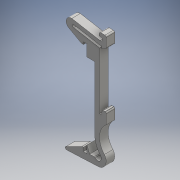
# Autodesk Inventor part: raspDinClipmmv3
Saved by Autodesk Inventor 2016 (Build 200138000, 138)
## iProperties
Created: 2016-08-27
Part Number: raspDinClipmmv3
Material: Generic
Document SubType Name: Modeling
Designer: Thetheos
Density: 1 g/cm^3
Appearance: Default
Author: Thetheos
Autodesk Inventor part; units mm, degrees
ref_plane "YZ Plane" through (0, 0, 0) normal (1, 0, 0) x (0, 1, 0)
ref_plane "XZ Plane" through (0, 0, 0) normal (0, 1, 0) x (-1, 0, 0)
ref_plane "XY Plane" through (0, 0, 0) normal (0, 0, 1) x (1, 0, 0)
sketch "Sketch1" plane through (0, 0, 0) normal (0, 1, 0) x (-1, 0, 0)
  arc A0 (-159.7794, 702.6597) -> (-160.5669, 701.8721) centre (-159.7794, 701.8721) ccw
  line L0 (-155.7462, 702.6597) -> (-155.7462, 704.2667)
  line L1 (-155.7462, 704.2667) -> (-153.5139, 704.2667)
  line L2 (-153.5139, 704.2667) -> (-153.5139, 702.7873)
  line L3 (-153.5139, 702.7873) -> (-152.617, 702.7873)
  arc A1 (-164.1836, 648.4268) -> (-160.5669, 657.8731) centre (-174.7114, 657.8731) ccw
  line L4 (-160.5669, 657.8731) -> (-160.5669, 701.8721)
  arc A2 (-160.1794, 645.8656) -> (-160.7583, 645.6139) centre (-160.1783, 645.0714) ccw
  arc A3 (-164.1836, 648.4268) -> (-160.7583, 645.6139) centre (-162.4137, 647.0901) ccw
  line L5 (-155.7462, 648) -> (-155.7462, 645.3343)
  line L6 (-155.7462, 645.3343) -> (-153.4959, 645.3343)
  line L7 (-153.4959, 645.3343) -> (-153.4959, 647.6194)
  arc A4 (-143.0505, 641.0266) -> (-142.8499, 642.7649) centre (-143.1474, 641.9185) ccw
  line L8 (-163.0481, 641.9081) -> (-143.0505, 641.0266)
  arc A5 (-166.527, 650.2868) -> (-163.0481, 641.9081) centre (-162.4027, 647.0877) ccw
  arc A6 (-166.527, 650.2868) -> (-167.6435, 666.7468) centre (-174.834, 657.9912) ccw
  line L9 (-166.9993, 673.5601) -> (-165.874, 673.5549)
  arc A7 (-165.1258, 673.0171) -> (-165.874, 673.5549) centre (-165.8807, 672.7563) ccw
  arc A8 (-163.8545, 670.6656) -> (-163.5889, 670.9316) centre (-163.8582, 670.9349) ccw
  line L10 (-163.5889, 706.0242) -> (-163.5889, 706.0613)
  line L11 (-163.5889, 706.0613) -> (-147.5669, 708.9022)
  arc A9 (-147.5669, 708.9022) -> (-147.8271, 710.4852) centre (-147.6086, 709.7082) ccw
  line L12 (-147.8271, 710.4852) -> (-163.5899, 707.6952)
  line L13 (-163.5899, 707.6952) -> (-164.9831, 707.6944)
  line L14 (-164.9831, 707.6944) -> (-164.9826, 706.5463)
  arc A10 (-165.396, 706.3271) -> (-164.9826, 706.5463) centre (-165.2521, 706.5552) ccw
  line L15 (-165.396, 706.3271) -> (-167.2486, 707.3943)
  arc A11 (-167.6628, 708.0983) -> (-167.2486, 707.3943) centre (-166.8615, 708.0959) ccw
  line L16 (-167.6628, 708.0983) -> (-167.6658, 713.6939)
  arc A12 (-166.8627, 714.4991) -> (-167.6658, 713.6939) centre (-166.8611, 713.6943) ccw
  line L17 (-166.8627, 714.4991) -> (-164.1837, 714.5007)
  arc A13 (-163.3795, 713.6976) -> (-164.1837, 714.5007) centre (-164.1848, 713.6954) ccw
  line L18 (-163.3795, 713.6976) -> (-163.3787, 712.3581)
  line L19 (-163.3787, 712.3581) -> (-165.5216, 711.9789)
  line L20 (-165.5216, 711.9789) -> (-165.5215, 711.7106)
  arc A14 (-165.5215, 711.7106) -> (-163.8456, 710.1095) centre (-163.9177, 711.7116) ccw
  line L21 (-163.8456, 710.1095) -> (-146.318, 713.1891)
  arc A15 (-144.6103, 707.1134) -> (-146.318, 713.1891) centre (-146.0422, 709.9888) ccw
  arc A16 (-152.617, 702.7873) -> (-152.2474, 702.8795) centre (-152.6236, 703.6003) ccw
  line L22 (-155.7462, 702.6597) -> (-155.7462, 700.1597)
  line L23 (-155.7462, 700.1597) -> (-156.9462, 700.1597)
  line L24 (-156.9462, 700.1597) -> (-157.7628, 702.6597)
  line L25 (-157.7628, 702.6597) -> (-159.7794, 702.6597)
  line L26 (-155.7462, 648) -> (-155.7462, 650)
  line L27 (-155.7462, 650) -> (-157.3545, 645.8656)
  line L28 (-157.3545, 645.8656) -> (-160.1794, 645.8656)
  line L29 (-144.6103, 707.1134) -> (-152.2474, 702.8795)
  line L30 (-152.5619, 647.6194) -> (-153.4959, 647.6194)
  line L31 (-163.8545, 670.6656) -> (-164.6545, 670.6656)
  arc A17 (-164.8084, 670.8401) -> (-164.6545, 670.6656) centre (-164.6322, 670.8403) ccw
  line L32 (-163.5889, 670.9316) -> (-163.5889, 706.0613)
  line L33 (-164.8084, 670.8401) -> (-165.1258, 673.0171)
  line L34 (-167.6435, 666.7468) -> (-167.6666, 672.6833)
  line L35 (-166.9993, 673.5601) -> (-167.2486, 673.5601)
  arc A18 (-167.2486, 673.5601) -> (-167.6666, 672.6833) centre (-166.547, 672.6876) ccw
  line L36 (-142.8499, 642.7649) -> (-152.5619, 647.6194)
  point P0 (-160.5669, 683.588)
  dimension "d2" = 43.999
  dimension "d6" = 2.5
  dimension "d7" = 1.2
  dimension "d8" = 2
  dimension "d18" = 0.8
  dimension "d20" = 2.2
  constraints: 74 end point, 38 point on circle, 19 centre point, 6 perpendicular, 5 horizontal, 2 tangent, 2 vertical
  measures "d2" distance of L4.start L4.end
  measures "d6" distance of L0.start L22.end
  measures "d7" distance of L22.end L23.end
  measures "d8" distance of L5.start L26.end
  measures "d18" distance of L31.start L31.end
  measures "d20" distance of L33.start L33.end
extrude "Extrusion1" add sketch "Sketch1" along normal blind 5.3
sketch "Sketch2" plane through (0, 0, 0) normal (0, -1, 0) x (1, 0, 0)
  line L0 (156.9462, 700.1597) -> (155.7462, 700.1597) projected
  line L1 (155.7462, 700.1597) -> (155.7462, 697.1597)
  line L2 (155.7462, 697.1597) -> (160.5669, 697.1597)
  line L3 (160.5669, 657.8731) -> (160.5669, 701.8721) projected
  line L4 (160.5669, 697.1597) -> (160.5783, 702.6397)
  line L5 (160.5783, 702.6397) -> (155.7462, 704.198)
  line L6 (155.7462, 704.198) -> (155.7462, 700.1597)
  point P0 (0, 0)
  dimension "d9" = 3
  constraints: 10 end point, 1 collinear, 1 perpendicular, 1 point on line, 1 vertical
  measures "d9" distance of L0.end L1.end
extrude "Extrusion2" add sketch "Sketch2" against normal blind 5.3
sketch "Sketch3" plane through (155.7462, 0, 704.2667) normal (-1, 0, 0) x (0, 0, 1)
  circle A0 centre (-4.5576, 2.65) radius 1.25
  line L0 (-7.107, 5.3) -> (0, 5.3) projected
  line L1 (0, 0) -> (-7.107, 0) projected
  point P0 (-704.2667, 0)
  dimension "d12" = 2.5
  dimension "d14" = 2.65
  dimension "d15" = 2.65
  constraints: 1 centre point
  measures "d12" diameter of A0
  measures "d14" distance from line of A0.centre L0
  measures "d15" distance from line of L1 A0.centre
extrude "Extrusion3" cut sketch "Sketch3" against normal blind 5
body "Solid1"
